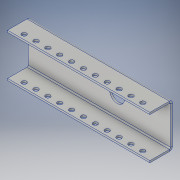
# Autodesk Inventor part: Side arm inner
Saved by Autodesk Inventor 2019 (Build 230136000, 136)
## iProperties
Created: 2018-11-07
Part Number: Side arm inner
Material: Aluminum 6061
Document SubType Name: Sheet Metal
Designer: woodk
Mass: 70.7409 g
Surface Area: 276.327 cm^2
Volume: 26.2003 cm^3
Density: 2.7 g/cm^3
Sheet Metal Rule: Haakon
Appearance: Aluminum - Flat
Author: woodk
Autodesk Inventor part; units mm, degrees
ref_plane "YZ Plane" through (0, 0, 0) normal (1, 0, 0) x (0, 1, 0)
ref_plane "XZ Plane" through (0, 0, 0) normal (0, 1, 0) x (-1, 0, 0)
ref_plane "XY Plane" through (0, 0, 0) normal (0, 0, 1) x (1, 0, 0)
sketch "Sketch1" plane through (0, 0, 0) normal (0, 0, 1) x (1, 0, 0)
  line L0 (0, 0) -> (152.4, 0)
  line L1 (152.4, 0) -> (152.4, 46.736)
  line L2 (152.4, 46.736) -> (0, 46.736)
  line L3 (0, 46.736) -> (0, 0)
  dimension "d0" = 152.4
  dimension "d1" = 46.736
  measures "d0" distance of L0.start L0.end
  measures "d1" distance of L2.end L0.start
extrude "Plate1" add sketch "Sketch1" along normal blind 2.032
sketch "Sketch2" plane through (0, 44.704, 0) normal (0, 1, 0) x (-1, 0, 0)
  line L0 (-152.4, 0) -> (0, 0)
  line L1 (0, 0) -> (0, 24.13)
  line L2 (0, 24.13) -> (-152.4, 24.13)
  line L3 (-152.4, 24.13) -> (-152.4, 0)
  constraints: 6 end point, 1 horizontal, 1 perpendicular, 1 vertical
edge flange "Flange1" height 24.13 angle 90 thickness 2.032 bend radius 1.27 thickness toward (0, 1, 0) relief tear relief width 2.032 relief depth 1.016 edges at (76.2, 46.736, 2.032) wall of the first edge with corners at (152.4, 44.704, 0) (0, 44.704, 0) (0, 44.704, 24.13) (152.4, 44.704, 24.13)
bend "Bend1"
corner "Corner1"
sketch "Sketch3" plane through (152.4, 2.032, 0) normal (0, -1, 0) x (1, 0, 0)
  line L0 (-152.4, 0) -> (0, 0)
  line L1 (0, 0) -> (0, 24.13)
  line L2 (0, 24.13) -> (-152.4, 24.13)
  line L3 (-152.4, 24.13) -> (-152.4, 0)
  constraints: 6 end point, 1 horizontal, 1 perpendicular, 1 vertical
edge flange "Flange2" height 24.13 angle 90 thickness 2.032 bend radius 1.27 thickness toward (0, -1, 0) relief tear relief width 2.032 relief depth 1.016 edges at (76.2, 0, 2.032) wall of the first edge with corners at (0, 2.032, 0) (152.4, 2.032, 0) (152.4, 2.032, 24.13) (0, 2.032, 24.13)
bend "Bend2"
corner "Corner2"
sketch "Sketch4" plane through (0, 46.736, 24.13) normal (0, 1, 0) x (1, 0, 0)
  line L0 (0, 0) -> (0, 20.828) projected
  line L1 (0, 24.13) -> (152.4, 24.13) projected
  point P0 (12.7, 5.08)
  dimension "d23" = 12.7
  dimension "d24" = 19.05
  measures "d23" distance from line of L0 point (12.7, 5.08)
  measures "d24" distance from line of point (12.7, 5.08) L1
hole "Hole1" at (12.7, 46.736, 19.05) direction (0, -1, 0) diameter 4.9784 end through all
pattern_linear "Rectangular Pattern1" count 11 spacing 12.7 along (1, 0, 0) of "Hole1"
sketch "Sketch5" plane through (0, 0, 0) normal (0, 0, -1) x (-1, 0, 0)
  line L0 (-152.4, 3.302) -> (-152.4, 43.434) projected
  point P0 (0, 0)
  point P1 (-95.25, 23.368)
  point P2 (-152.4, 23.368)
  dimension "d35" = 57.15
  constraints: 1 horizontal alignment, 1 midpoint
  measures "d35" distance from line of L0 point (-95.25, 23.368)
hole "Hole2" at (95.25, 23.368, 0) direction (0, 0, 1) diameter 15.875 end through all
equation "\"d30\" = Thickness"
equation "\"d41\" = Thickness"
equation "\"d2\" = Thickness"
equation "\"d3\" = BendReliefWidth"
equation "\"d4\" = BendReliefDepth"
equation "\"d5\" = MinimumRemnant"
equation "\"d6\" = TransitionRadius"
equation "\"d9\" = BendRadius"
equation "\"d10\" = CornerReliefSize"
equation "\"d11\" = GapSize"
equation "\"d12\" = JacobiRadiusSize"
equation "\"d13\" = BendReliefWidth"
equation "\"d14\" = BendReliefDepth"
equation "\"d15\" = MinimumRemnant"
equation "\"d16\" = TransitionRadius"
equation "\"d19\" = BendRadius"
equation "\"d20\" = CornerReliefSize"
equation "\"d21\" = GapSize"
equation "\"d22\" = JacobiRadiusSize"
equation "\"BendReliefWidth\" = Thickness"
equation "\"BendReliefDepth\" = 0.5 * Thickness"
equation "\"CornerReliefSize\" = 4 * Thickness"
equation "\"MinimumRemnant\" = 2 * Thickness"
equation "\"TransitionRadius\" = BendRadius"
equation "\"JacobiRadiusSize\" = BendRadius"
equation "\"GapSize\" = Thickness"
equation "\"Thickness\" = 2.032"
equation "\"BendRadius\" = 1.27"
body "Solid1"
